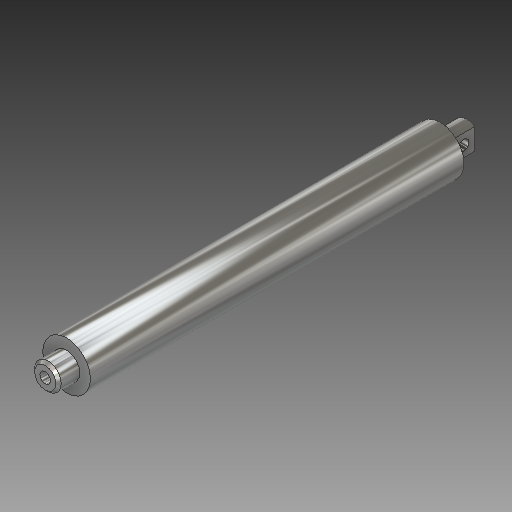
# Autodesk Inventor part: cylinder body
Saved by Autodesk Inventor 2017 SP1 (Build 210196100, 196)
## iProperties
Created: 2018-01-27
Part Number: cylinder body
Material: Generic
Document SubType Name: Modeling
Designer: Ben
Density: 1 g/cm^3
Appearance: Chrome - Polished
Mass: 140.336 g
Surface Area: 255.724 cm^2
Volume: 140.336 cm^3
Author: Ben
Autodesk Inventor part; units mm, degrees
ref_plane "YZ Plane" through (0, 0, 0) normal (1, 0, 0) x (0, 1, 0)
ref_plane "XZ Plane" through (0, 0, 0) normal (0, 1, 0) x (-1, 0, 0)
ref_plane "XY Plane" through (0, 0, 0) normal (0, 0, 1) x (1, 0, 0)
sketch "Sketch1" plane through (0, 0, 0) normal (0, 0, 1) x (1, 0, 0)
  circle A0 centre (0, 0) radius 14.1986
  dimension "d0" = 28.3972
  constraints: 1 centre point, 1 coincident
  measures "d0" diameter of A0
extrude "Extrusion1" add sketch "Sketch1" along normal mid plane 222.25
sketch "Sketch2" plane through (0, 0, -111.125) normal (0, 0, -1) x (-1, 0, 0)
  arc A0 (4.7625, 6.35) -> (-4.7625, 6.35) centre (0, 0) ccw
  arc A1 (-4.7625, -6.35) -> (4.7625, -6.35) centre (0, 0) ccw
  line L0 (-4.7625, 6.35) -> (-4.7625, -6.35)
  line L1 (4.7625, 6.35) -> (4.7625, -6.35)
  line L2 (4.7625, 0) -> (-4.7625, 0) construction
  dimension "d3" = 9.525
  dimension "d4" = 7.9375
  constraints: 6 end point, 4 point on circle, 3 coincident, 3 midpoint, 2 centre point, 1 concentric, 1 parallel, 1 vertical
  measures "d3" distance of L2.start L2.end
  measures "d4" radius of A0
extrude "Extrusion2" add sketch "Sketch2" along normal blind 15.875
sketch "Sketch3" plane through (4.7625, -6.35, -111.125) normal (1, 0, 0) x (0, 0, -1)
  line L0 (15.875, 12.7) -> (15.875, 0) construction
  line L1 (15.875, 6.35) -> (0, 6.35) construction
  line L2 (0, -7.8486) -> (0, 20.5486) construction
  circle A0 centre (9.271, 6.35) radius 3.175
  point P0 (-111.125, 6.35)
  dimension "d7" = 6.604
  dimension "d8" = 6.35
  constraints: 2 end point, 2 midpoint, 1 centre point, 1 point on line
  measures "d7" distance from line of L0 A0.centre
  measures "d8" diameter of A0
extrude "Extrusion3" cut sketch "Sketch3" against normal through all
sketch "Sketch4" plane through (0, 0, 111.125) normal (0, 0, 1) x (1, 0, 0)
  circle A0 centre (0, 0) radius 7.9375
  dimension "d11" = 15.875
  constraints: 1 centre point, 1 coincident
  measures "d11" diameter of A0
extrude "Extrusion4" add sketch "Sketch4" along normal blind 12.7
chamfer "Chamfer1" distance 1.5875 angle 45 1 edges at (-7.9375, 0, 123.825)
sketch "Sketch5" plane through (0, 0, 123.825) normal (0, 0, 1) x (1, 0, 0)
  circle A0 centre (0, 0) radius 3.175
  dimension "d17" = 6.35
  constraints: 1 centre point, 1 coincident
  measures "d17" diameter of A0
extrude "Extrusion5" cut sketch "Sketch5" against normal blind 152.4
body "Solid1"
